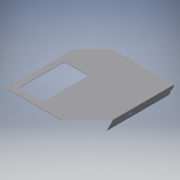
# Autodesk Inventor part: sheetblack
Saved by Autodesk Inventor 2016 (Build 200138000, 138)
## iProperties
Created: 2018-11-08
Part Number: sheetblack
Material: Generic
Document SubType Name: Sheet Metal
Designer: hovm
Density: 1 g/cm^3
Sheet Metal Rule: Default_mm
Appearance: Default
Author: hovm
Autodesk Inventor part; units mm, degrees
ref_plane "YZ Plane" through (0, 0, 0) normal (1, 0, 0) x (0, 1, 0)
ref_plane "XZ Plane" through (0, 0, 0) normal (0, 1, 0) x (-1, 0, 0)
ref_plane "XY Plane" through (0, 0, 0) normal (0, 0, 1) x (1, 0, 0)
sketch "Sketch1" plane through (0, 0, 0) normal (0, 0, 1) x (1, 0, 0)
  line L0 (-29.5815, 53.7121) -> (-29.5815, 355.2879)
  line L1 (-329.5815, 355.5) -> (-54.5815, 355.5)
  line L2 (-329.5815, 53.5) -> (-54.5815, 53.5)
  line L3 (-310.5815, 334.5) -> (-310.5815, 74.5)
  line L4 (-29.5815, 355.5) -> (-310.5815, 355.5)
  line L5 (-310.5815, 355.5) -> (-310.5815, 53.5)
  line L6 (-310.5815, 53.5) -> (-29.5815, 53.5)
  line L7 (-29.5815, 53.5) -> (-29.5815, 355.5)
  point P0 (0, 0)
extrude "Plate1" add sketch "Sketch1" along normal blind 1
sketch "Sketch2" plane through (-29.5815, 53.5, 0) normal (1, 0, 0) x (0, 1, 0)
  line L0 (302, 0) -> (0, 0)
  line L1 (0, 0) -> (0, -21)
  line L2 (0, -21) -> (302, -21)
  line L3 (302, -21) -> (302, 0)
  constraints: 6 end point, 1 horizontal, 1 perpendicular, 1 vertical
edge flange "Flange1" height 22 angle 90 thickness 1 bend radius 1 thickness toward (1, 0, 0) relief tear relief width 1 relief depth 0.5 edges at (-29.5815, 204.5, 0) wall of the first edge with corners at (-29.5815, 355.5, 0) (-29.5815, 53.5, 0) (-29.5815, 53.5, -21) (-29.5815, 355.5, -21)
bend "Bend1"
corner "Corner1"
chamfer "Corner Chamfer1" distance 18 angle 45 1 edges at (-29.0815, 355.5, -21)
chamfer "Corner Chamfer2" distance 18 angle 45 1 edges at (-29.0815, 53.5, -21)
chamfer "Corner Chamfer3" distance 6 angle 45 2 edges at (-310.5815, 355.5, 0.5) (-310.5815, 53.5, 0.5)
sketch "Sketch3" plane through (0, 0, 1) normal (0, 0, 1) x (1, 0, 0)
  line L0 (-310.5815, 59.5) -> (-310.5815, 349.5) projected
  line L1 (-304.5815, 355.5) -> (-30.5815, 355.5) projected
  line L2 (-304.5815, 53.5) -> (-30.5815, 53.5) projected
  point P0 (0, 0)
  point P1 (-77.5815, 345.5)
  point P2 (-167.5815, 345.5)
  point P3 (-257.5815, 345.5)
  point P4 (-300.5815, 344.5)
  point P5 (-300.5815, 204.5)
  point P6 (-300.5815, 64.5)
  point P7 (-257.5815, 63.5)
  point P8 (-167.5815, 63.5)
  point P9 (-77.5815, 63.5)
  point P10 (-310.5815, 204.5)
  point P11 (-167.5815, 355.5)
  dimension "d20" = 90
  dimension "d21" = 90
  dimension "d22" = 10
  dimension "d23" = 10
  dimension "d24" = 140
  dimension "d25" = 140
  dimension "d26" = 10
  constraints: 6 vertical alignment, 5 horizontal alignment, 2 midpoint
  measures "d20" distance of point (-77.581, 345.5) point (-167.581, 345.5)
  measures "d21" distance of point (-167.581, 345.5) point (-257.581, 345.5)
  measures "d22" distance from line of L1 point (-77.581, 345.5)
  measures "d23" distance from line of L2 point (-77.581, 63.5)
  measures "d24" distance of point (-300.581, 204.5) point (-300.581, 344.5)
  measures "d25" distance of point (-300.581, 64.5) point (-300.581, 204.5)
  measures "d26" distance from line of point (-300.581, 64.5) L0
hole "Hole1" at (-77.5815, 345.5, 1) at (-167.5815, 345.5, 1) at (-257.5815, 345.5, 1) at (-300.5815, 344.5, 1) at (-300.5815, 204.5, 1) at (-300.5815, 64.5, 1) at (-257.5815, 63.5, 1) at (-167.5815, 63.5, 1) at (-77.5815, 63.5, 1) direction (0, 0, -1) diameter 4 depth 1 tip angle 118
sketch "Sketch4" plane through (-28.5815, 53.5, -1) normal (1, 0, 0) x (0, 0, -1)
  line L0 (20, 284) -> (20, 18) projected
  point P0 (-1, -53.5)
  point P1 (10, 291)
  point P2 (10, 151)
  point P3 (10, 11)
  point P4 (20, 151)
  dimension "d34" = 10
  dimension "d35" = 140
  dimension "d36" = 140
  constraints: 2 vertical alignment, 1 horizontal alignment, 1 midpoint
  measures "d34" distance from line of L0 point (10, 291)
  measures "d35" distance of point (10, 291) point (10, 151)
  measures "d36" distance of point (10, 151) point (10, 11)
hole "Hole2" at (-28.5815, 344.5, -11) at (-28.5815, 204.5, -11) at (-28.5815, 64.5, -11) direction (-1, 0, 0) diameter 4 depth 1 tip angle 118
sketch "Sketch5" plane through (0, 0, 1) normal (0, 0, 1) x (1, 0, 0)
  line L0 (-288.5815, 83.5) -> (-288.5815, 325.5) projected
  line L1 (-329.5815, 74.5) -> (-54.5815, 74.5) projected
  line L2 (-204.5815, 234.5) -> (-288.5815, 234.5)
  line L3 (-288.5815, 234.5) -> (-288.5815, 74.5)
  line L4 (-288.5815, 74.5) -> (-204.5815, 74.5)
  line L5 (-204.5815, 74.5) -> (-204.5815, 234.5)
  point P0 (0, 0)
  dimension "d44" = 84
  dimension "d45" = 160
  constraints: 8 end point, 2 parallel, 1 collinear, 1 horizontal, 1 perpendicular, 1 point on line
  measures "d44" distance of L2.start L2.end
  measures "d45" distance of L4.end L2.start
extrude "Cut1" cut sketch "Sketch5" against normal blind 1
fillet "Corner Round1" radius 6 4 edges at (-204.5815, 234.5, 0.5) (-288.5815, 234.5, 0.5) (-204.5815, 74.5, 0.5) (-288.5815, 74.5, 0.5)
sketch "Sketch6" plane through (0, 0, 1) normal (0, 0, 1) x (1, 0, 0)
  line L0 (-304.5815, 355.5) -> (-30.5815, 355.5) projected
  line L1 (-310.5815, 349.5) -> (-310.5815, 59.5) projected
  point P0 (0, 0)
  point P1 (-280.5815, 325.5)
  dimension "d49" = 30
  dimension "d50" = 30
  measures "d49" distance from line of point (-280.581, 325.5) L0
  measures "d50" distance from line of L1 point (-280.581, 325.5)
hole "Hole3" at (-280.5815, 325.5, 1) direction (0, 0, -1) diameter 8 depth 1 tip angle 118
equation "\"d21\" = d20"
equation "\"d25\" = d24"
equation "\"d32\" = Thickness"
equation "\"d36\" = d35"
equation "\"d42\" = Thickness"
equation "\"d46\" = Thickness"
equation "\"d56\" = Thickness"
equation "\"d1\" = BendReliefWidth"
equation "\"d2\" = BendReliefDepth"
equation "\"d3\" = MinimumRemnant"
equation "\"d4\" = BendRadius"
equation "\"d7\" = BendRadius"
equation "\"d8\" = CornerReliefSize"
equation "\"d9\" = GapSize"
equation "\"d10\" = JacobiRadiusSize"
equation "\"BendRadius\" = Thickness"
equation "\"BendReliefWidth\" = Thickness"
equation "\"BendReliefDepth\" = 0.5 * Thickness"
equation "\"CornerReliefSize\" = 4 * Thickness"
equation "\"MinimumRemnant\" = 2 * Thickness"
equation "\"TransitionRadius\" = BendRadius"
equation "\"JacobiRadiusSize\" = BendRadius"
equation "\"GapSize\" = Thickness"
equation "\"d0\" = BendRadius"
equation "\"Thickness\" = 1"
body "Solid1"
